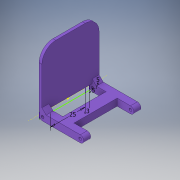
# Autodesk Inventor part: Mouth-Height-Lever-front
Saved by Autodesk Inventor 2018.3 (Build 223284000, 284)
## iProperties
Created: 2018-05-17
Part Number: Mouth-Height-Lever-front
Material: Generisch
Document SubType Name: Modeling
Designer: JochenAlt
Density: 1 g/cm^3
Appearance: Violett
Author: JochenAlt
Autodesk Inventor part; units mm, degrees
ref_plane "YZ Plane" through (0, 0, 0) normal (1, 0, 0) x (0, 1, 0)
ref_plane "XZ Plane" through (0, 0, 0) normal (0, 1, 0) x (-1, 0, 0)
ref_plane "XY Plane" through (0, 0, 0) normal (0, 0, 1) x (1, 0, 0)
sketch "Skizze1" plane through (0, 0, 0) normal (1, 0, 0) x (0, 1, 0)
  line L0 (0, 3.3571) -> (0, -3.6429) construction
  line L1 (-28.7, 0) -> (28.7, 0) construction
  line L2 (20.5, 2.3571) -> (15.5, 2.3571)
  line L3 (15.5, 2.3571) -> (15.5, -2.6429)
  line L4 (15.5, -2.6429) -> (20.5, -2.6429)
  line L5 (20.5, -2.6429) -> (20.5, 2.3571)
  line L6 (-15.5, 2.3571) -> (-20.5, 2.3571)
  line L7 (-20.5, 2.3571) -> (-20.5, -2.6429)
  line L8 (-20.5, -2.6429) -> (-15.5, -2.6429)
  line L9 (-15.5, -2.6429) -> (-15.5, 2.3571)
  line L10 (12.5, 2.3571) -> (-12.5, 2.3571)
  line L11 (-12.5, 2.3571) -> (-12.5, -2.6429)
  line L12 (-12.5, -2.6429) -> (12.5, -2.6429)
  line L13 (12.5, -2.6429) -> (12.5, 2.3571)
  line L14 (15.5, 2.3571) -> (12.5, 2.3571)
  line L15 (15.5, -2.6429) -> (12.5, -2.6429)
  line L16 (-12.5, 2.3571) -> (-15.5, 2.3571)
  line L17 (-12.5, -2.6429) -> (-15.5, -2.6429)
  point P0 (0, 0)
  dimension "d0" = 5
  dimension "d1" = 5
  dimension "d2" = 25
  dimension "d3" = 3
  constraints: 32 end point, 6 horizontal, 6 parallel, 3 perpendicular, 1 collinear, 2 other
  measures "d0" distance of L3.end L4.end
  measures "d1" distance of L4.end L2.start
  measures "d2" distance of L11.end L12.end
  measures "d3" distance between parallel lines of L3 L13
extrude "Extrusion1" add sketch "Skizze1" along normal blind 12 contours L5 L4 L3 L2 | L9 L8 L7 L6
extrude "Extrusion2" add sketch "Skizze1" along normal blind 8 from surface at 12
extrude "Extrusion3" add sketch "Skizze1" along normal blind 12 from surface at 20 contours L5 L4 L3 L2 | L9 L8 L7 L6
fillet "Rundung1" radius 2.5 6 edges at (32, 18, 2.3571) (32, 18, -2.6429) (32, -18, 2.3571) (32, -18, -2.6429) (0, 18, -2.6429) (0, -18, -2.6429)
sketch "Skizze2" plane through (2.5, -20.5, -2.6429) normal (0, -1, 0) x (1, 0, 0)
  circle A0 centre (27, 2.5) radius 1
  circle A1 centre (0, 2.5) radius 1
  arc A2 (27, 0) -> (27, 5) centre (27, 2.5) ccw projected
  arc A3 (-2.5, 2.5) -> (0, 0) centre (0, 2.5) ccw projected
  point P0 (-2.5, 2.6429)
  point P1 (0, 5)
  dimension "d11" = 2
  constraints: 2 centre point, 2 concentric, 1 equal radius
  measures "d11" diameter of A0
extrude "Extrusion4" cut sketch "Skizze2" against normal through all
sketch "Skizze3" plane through (0, -15, 2.3571) normal (0, 0, 1) x (1, 0, 0)
  line L0 (0, -0.5) -> (0, -5.5) projected
  line L1 (29.5, 35.5) -> (0, 35.5) projected
  line L2 (0, -5.5) -> (2, -5.5)
  line L3 (2, -5.5) -> (2, 35.5)
  line L4 (2, 35.5) -> (0, 35.5)
  line L5 (0, 35.5) -> (0, -5.5)
  point P0 (0, 15)
  dimension "d14" = 2
  constraints: 8 end point, 2 parallel, 1 horizontal, 1 perpendicular, 1 point on line
  measures "d14" distance of L0.end L2.end
extrude "Extrusion5" add sketch "Skizze3" along normal blind 40
fillet "Rundung2" radius 10 2 edges at (1, 20.5, 42.3571) (1, -20.5, 42.3571)
chamfer "Fase1" distance 3 angle 45 2 edges at (2, 18, 2.3571) (2, -18, 2.3571)
equation "\"d10\" = 0.5 * d1"
